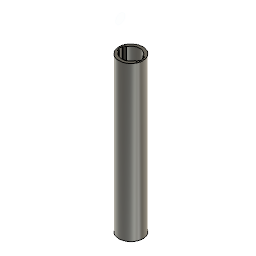
Body (Autodesk Fusion 360 design; units mm, degrees)
part number: 2026-02-03-16-03-13-977
Autodesk Fusion 360 part; units mm, degrees
sketch "Sketch1" plane through (0, 0, 0) normal (0, 0, 1) x (1, 0, 0)
  circle A0 centre (0, 0) radius 12.5
  dimension "d1" = 25
  constraint coincident A0.centre origin
  measures "d1" diameter of A0
extrude "Extrude1" add sketch "Sketch1" along normal blind 160
sketch "Sketch3" plane through (0, 0, 160) normal (0, 0, 1) x (-1, 0, 0)
  circle A0 centre (0, 0) radius 12.5
  circle A1 centre (0, 0) radius 9.5
  dimension "d4" = 19
  constraint concentric A0 A1
  measures "d4" diameter of A1
extrude "Extrude2" cut sketch "Sketch3" against normal blind 1000 contours A1
sketch "Sketch4" plane through (0, 0, 160) normal (0, 0, -1) x (1, 0, 0)
  circle A0 centre (0, -30) radius 12.5
  circle A1 centre (0, -30) radius 9.25
  dimension "d12" = 18.5
  constraint concentric A0 A1
  measures "d12" diameter of A1
sketch "Sketch7" plane through (0, 0, 171) normal (0, 0, 1) x (-1, 0, 0)
  circle A0 centre (30, 0) radius 6.2204
  circle A1 centre (30, 0) radius 5
  constraint concentric A0 A1
sketch "Sketch8" plane through (0, 0, 171) normal (0, 0, 1) x (-1, 0, 0)
  circle A0 centre (30, 0) radius 5
  circle A1 centre (30, 0) radius 6.2204
  line L0 (26, -15) -> (14, -15)
  circle A2 centre (20, -15) radius 6
  line L1 (26, -20) -> (21, -20)
  line L2 (21, -10) -> (26, -10)
  line L3 (26, -10) -> (26, -20)
  constraint horizontal L0
  constraint coincident L0.start A2
  constraint coincident L0.end A2
  constraint horizontal L1
  constraint horizontal L2
  constraint vertical L3
sketch "Sketch9" plane through (-26, 0, 0) normal (-1, 0, 0) x (0, -1, 0)
  circle A0 centre (-15, 171) radius 5
sketch "Sketch10" plane through (-26, 0, 0) normal (-1, 0, 0) x (0, -1, 0)
  circle A0 centre (-15, 171) radius 4
sketch "Sketch11" plane through (0, 0, 160) normal (0, 0, 1) x (-1, 0, 0)
  circle A0 centre (0, 0) radius 9.5
  circle A1 centre (0, 0) radius 12.5
  line L0 (11, 2) -> (-11, 2)
  line L1 (-11, 2) -> (-11, -2)
  line L2 (-11, -2) -> (11, -2)
  line L3 (11, -2) -> (11, 2)
  line L4 (10, -4) -> (-10, -4)
  line L5 (-10, -4) -> (-10, 4)
  line L6 (-10, 4) -> (10, 4)
  line L7 (10, 4) -> (10, -4)
  constraint horizontal L0
  constraint vertical L1
  constraint horizontal L2
  constraint vertical L3
  constraint horizontal L4
  constraint vertical L5
  constraint horizontal L6
  constraint vertical L7
extrude "Extrude7" cut sketch "Sketch11" against normal blind 155 contours A0 L0 L2 L7 | A0 L0 L6 L7 | A0 L2 L4 L7 | L0 L2 L3 L7 | A0 L0 L5 L6 | A0 L0 L2 L5 | A0 L2 L4 L5 | L0 L1 L2 L5
sketch "Sketch12" plane through (0, 0, 160) normal (0, 0, 1) x (-1, 0, 0)
  line L0 (11, -2) -> (10, -2)
  arc A0 (8.6168, 4) -> (-8.6168, 4) centre (0, 0) ccw
  line L1 (-10, -2) -> (-11, -2)
  line L2 (-11, -2) -> (-11, 2)
  line L3 (-11, 2) -> (-10, 2)
  line L4 (10, 2) -> (11, 2)
  line L5 (11, 2) -> (11, -2)
  circle A1 centre (0, 0) radius 12.5
  line L6 (10.9, -1.9) -> (-10.9, -1.9)
  line L7 (-10.9, -1.9) -> (-10.9, 1.9)
  line L8 (-10.9, 1.9) -> (10.9, 1.9)
  line L9 (10.9, 1.9) -> (10.9, -1.9)
  line L10 (10, -3) -> (-10, -3)
  line L11 (-10, -3) -> (-10, 3)
  line L12 (-10, 3) -> (10, 3)
  line L13 (10, 3) -> (10, -3)
  line L14 (-8.6168, -4) -> (-10, -4)
  line L15 (-10, -4) -> (-10, -2)
  line L16 (-10, 2) -> (-10, 4)
  line L17 (-10, 4) -> (-8.6168, 4)
  line L18 (8.6168, 4) -> (10, 4)
  line L19 (10, 4) -> (10, 2)
  line L20 (10, -2) -> (10, -4)
  line L21 (10, -4) -> (8.6168, -4)
  arc A2 (-8.6168, -4) -> (8.6168, -4) centre (0, 0) ccw
  constraint horizontal L6
  constraint vertical L7
  constraint horizontal L8
  constraint vertical L9
  constraint horizontal L10
  constraint vertical L11
  constraint horizontal L12
  constraint vertical L13
sketch "Sketch13" plane through (0, -1.9, 0) normal (0, -1, 0) x (1, 0, 0)
  line L0 (37.9, 160) -> (16.1, 160)
  line L1 (16.1, 160) -> (16.1, 0)
  line L2 (16.1, 0) -> (37.9, 0)
  line L3 (37.9, 0) -> (37.9, 160)
  line L4 (18, 158) -> (36, 158)
  line L5 (36, 158) -> (36, 16)
  line L6 (36, 16) -> (18, 16)
  line L7 (18, 16) -> (18, 158)
  constraint horizontal L4
  constraint vertical L5
  constraint horizontal L6
  constraint vertical L7
sketch "Sketch14" plane through (0, -1.9, 0) normal (0, -1, 0) x (1, 0, 0)
  line L0 (16, 0) -> (19.1, 0)
  line L1 (19.1, 0) -> (19.1, 5.1)
  line L2 (19.1, 5.1) -> (16, 5.1)
  line L3 (16, 5.1) -> (16, 0)
  line L4 (38, 0) -> (34.9, 0)
  line L5 (34.9, 0) -> (34.9, 5.1)
  line L6 (34.9, 5.1) -> (38, 5.1)
  line L7 (38, 5.1) -> (38, 0)
  constraint horizontal L0
  constraint vertical L1
  constraint horizontal L2
  constraint vertical L3
  constraint horizontal L4
  constraint vertical L5
  constraint horizontal L6
  constraint vertical L7
sketch "Sketch15" plane through (0, 0, 0) normal (0, 0, -1) x (1, 0, 0)
  line L0 (19.1, 1.9) -> (19.1, -1.9)
  line L1 (19.1, -1.9) -> (34.9, -1.9)
  line L2 (34.9, -1.9) -> (34.9, 1.9)
  line L3 (34.9, 1.9) -> (19.1, 1.9)
  circle A0 centre (27, 0) radius 7.9
  circle A1 centre (27, 0) radius 7.6941
  constraint tangent L0 A0
  constraint concentric A0 A1
